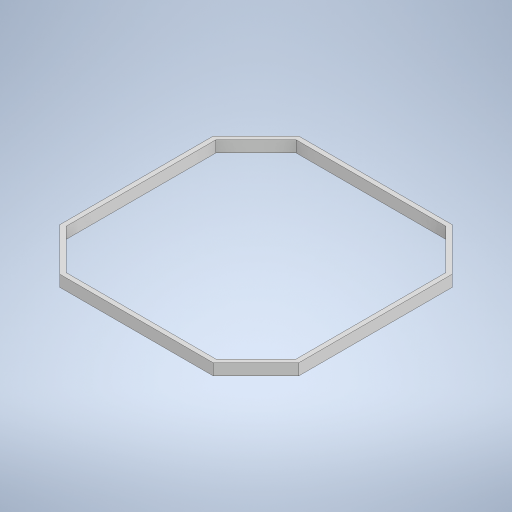
# Autodesk Inventor part: 팔각형 OV-PAM 5패턴 층 한개 부피 구하기 0도 - 수정
Saved by Autodesk Inventor 2024 (Build 280153000, 153)
## iProperties
Created: 2023-06-20
Part Number: 팔각형 OV-PAM 5패턴 층 한개 부피 구하기 0도 - 수정
Material: 일반
Document SubType Name: Modeling
Designer: jsw
Density: 1 g/cm^3
Appearance: 기본값
Mass: 0.236847 g
Surface Area: 8.28964 cm^2
Volume: 0.236847 cm^3
Author: jsw
Autodesk Inventor part; units mm, degrees
ref_plane "YZ Plane" through (0, 0, 0) normal (1, 0, 0) x (0, 1, 0)
ref_plane "XZ Plane" through (0, 0, 0) normal (0, 1, 0) x (-1, 0, 0)
ref_plane "XY Plane" through (0, 0, 0) normal (0, 0, 1) x (1, 0, 0)
sketch "스케치1" plane through (0, 0, 0) normal (0, 1, 0) x (-1, 0, 0)
  line L0 (-32.5919, 13.5) -> (-13.5, 32.5919)
  line L1 (-13.5, 32.5919) -> (13.5, 32.5919)
  line L2 (13.5, 32.5919) -> (32.5919, 13.5)
  line L3 (32.5919, 13.5) -> (32.5919, -13.5)
  line L4 (32.5919, -13.5) -> (13.5, -32.5919)
  line L5 (13.5, -32.5919) -> (-13.5, -32.5919)
  line L6 (-13.5, -32.5919) -> (-32.5919, -13.5)
  line L7 (-32.5919, -13.5) -> (-32.5919, 13.5)
  line L8 (21.0459, 13.5) -> (21.0459, -13.5)
  line L9 (-21.0459, -13.5) -> (-21.0459, 13.5)
  line L10 (13.5, -21.0459) -> (-13.5, -21.0459)
  line L11 (-13.5, 21.0459) -> (13.5, 21.0459)
  line L12 (13.5, -21.0459) -> (21.0459, -13.5)
  line L13 (21.0459, 13.5) -> (13.5, 21.0459)
  line L14 (-13.5, 21.0459) -> (-21.0459, 13.5)
  line L15 (-21.0459, -13.5) -> (-13.5, -21.0459)
  point P0 (0, 0)
  point P1 (0, 0)
  point P2 (0, 21.0459)
  point P3 (0, -32.5919)
  dimension "d0" = 27
  dimension "d1" = 11.546
  dimension "d2" = 11.546
  dimension "d3" = 11.546
  dimension "d4" = 11.546
  constraints: 32 end point, 4 horizontal alignment, 4 vertical alignment, 3 horizontal, 2 midpoint, 2 vertical, 1 coincident, 17 other
  measures "d0" distance of L2.end L3.end
  measures "d1" distance between parallel lines of L8 L3
  measures "d2" distance from line of L10 point (0, -32.592)
  measures "d3" distance between parallel lines of L7 L9
  measures "d4" distance between parallel lines of L1 L11
extrude "돌출1" add sketch "스케치1" along normal blind 2 contours L8 L12 L10 L15 L9 L14 L11 L13
shell "쉘1" thickness 0.8 removed faces 2 at (7.0153, 0, 4.5) at (7.0153, 2, 4.5)
